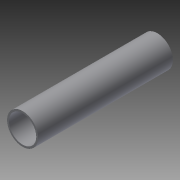
# Autodesk Inventor part: CNC-Y-axis- slider tube
Saved by Autodesk Inventor 2015 (Build 190159000, 159)
## iProperties
Created: 2015-06-12
Part Number: CNC-Y-axis- slider tube
Material: Generic
Document SubType Name: Modeling
Designer: Bangladesh
Density: 1 g/cm^3
Appearance: Default
Author: Bangladesh
Autodesk Inventor part; units mm, degrees
ref_plane "YZ Plane" through (0, 0, 0) normal (1, 0, 0) x (0, 1, 0)
ref_plane "XZ Plane" through (0, 0, 0) normal (0, 1, 0) x (-1, 0, 0)
ref_plane "XY Plane" through (0, 0, 0) normal (0, 0, 1) x (1, 0, 0)
sketch "Sketch1" plane through (0, 0, 0) normal (0, 0, 1) x (1, 0, 0)
  circle A0 centre (0, 0) radius 10.2235
  dimension "d0" = 20.447
  constraints: 1 centre point, 1 coincident
  measures "d0" diameter of A0
extrude "Extrusion1" add sketch "Sketch1" along normal mid plane 88.9
sketch "Sketch2" plane through (0, 0, 44.45) normal (0, 0, 1) x (1, 0, 0)
  circle A0 centre (0, 0) radius 5.0469
  constraints: 1 centre point, 1 coincident
hole "Hole1" at (0, 0, 44.45) direction (0, 0, -1) diameter 18 end through all
body "Solid1"
